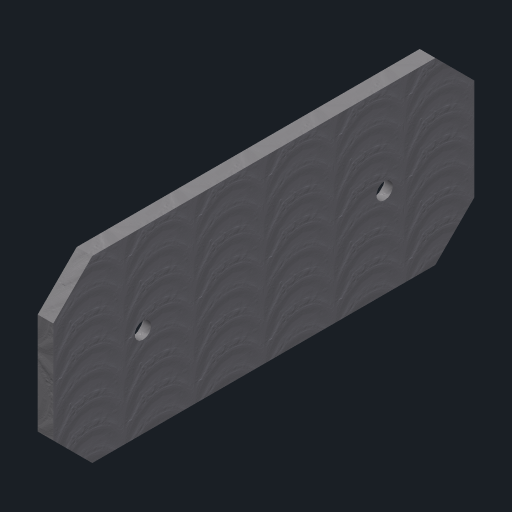
# Autodesk Inventor part: CAJA
Saved by Autodesk Inventor 2024.3 (Build 283343000, 343)
## iProperties
Created: 2024-06-29
Part Number: CAJA
Material: Steel, Mild, Welded
Document SubType Name: Modeling
Designer: Niler
Density: 7.85 g/cm^3
Appearance: Weld - Steel Mild
Author: Niler
Autodesk Inventor part; units mm, degrees
ref_plane "YZ Plane" through (0, 0, 0) normal (1, 0, 0) x (0, 1, 0)
ref_plane "XZ Plane" through (0, 0, 0) normal (0, 1, 0) x (-1, 0, 0)
ref_plane "XY Plane" through (0, 0, 0) normal (0, 0, 1) x (1, 0, 0)
sketch "Sketch1" plane through (0, 0, 0) normal (1, 0, 0) x (0, 1, 0)
  line L0 (-57.5, 135) -> (57.5, 135)
  line L1 (57.5, 135) -> (57.5, -135)
  line L2 (57.5, -135) -> (-57.5, -135)
  line L3 (-57.5, -135) -> (-57.5, 135)
  line L4 (-57.5, 135) -> (57.5, -135) construction
  line L5 (57.5, 135) -> (-57.5, -135) construction
  circle A0 centre (0, 77.5) radius 5.3
  circle A1 centre (0, -77.5) radius 5.3
  circle A2 centre (0, 0) radius 5.3
  line L6 (0, 77.5) -> (0, -77.5) construction
  line L7 (51.5, -129) -> (51.5, 129)
  line L8 (51.5, 129) -> (-51.5, 129)
  line L9 (-51.5, 129) -> (-51.5, -129)
  line L10 (-51.5, -129) -> (51.5, -129)
  dimension "d0" = 155
  dimension "d1" = 10.6
  dimension "d2" = 270
  dimension "d3" = 115
  dimension "d4" = 6
  constraints: 22 end point, 4 parallel, 3 centre point, 3 midpoint, 2 equal radius, 2 perpendicular, 2 vertical alignment, 1 coincident, 1 horizontal, 1 vertical, 3 other
  measures "d0" distance of L6.end L6.start
  measures "d1" diameter of A0
  measures "d2" distance between parallel lines of L2 L0
  measures "d3" distance of L0.start L0.end
  measures "d4" distance between parallel lines of L1 L7
extrude "Extrusion1" add sketch "Sketch1" along normal blind 10 contours L0 L1 L2 L3 | A2 | L10 L9 L8 L7
chamfer "Chamfer2" distance 25 angle 45 4 edges at (5, 57.5, -135) (5, -57.5, -135) (5, -57.5, 135) (5, 57.5, 135)
sketch "Sketch11" plane through (0, 0, 0) normal (-1, 0, 0) x (0, 0, 1)
  circle A0 centre (-77.5, 0) radius 5.3 projected
  circle A1 centre (77.5, 0) radius 5.3 projected
  circle A2 centre (-77.5, 0) radius 11.15
  circle A3 centre (77.5, 0) radius 11.15
  point P0 (0, 0)
  dimension "d41" = 22.3
  constraints: 2 centre point, 2 coincident, 1 equal radius
  measures "d41" diameter of A2
extrude "Extrusion10" cut sketch "Sketch11" against normal blind 5 contours A0 | A1 | A2 | A3
sketch "Sketch12" plane through (0, 0, 0) normal (-1, 0, 0) x (0, 0, 1)
  circle A0 centre (0, -15) radius 9.65
  point P0 (0, 0)
  dimension "d44" = 15
  dimension "d45" = 19.3
  constraints: 1 centre point, 1 vertical alignment
  measures "d44" distance of A0.centre point (0, 0)
  measures "d45" diameter of A0
extrude "Extrusion11" cut sketch "Sketch12" against normal blind 5
sketch "Sketch13" plane through (5, -15, 0) normal (-1, 0, 0) x (0, 0, 1)
  circle A0 centre (0, 0) radius 9.65 projected
  circle A1 centre (0, 0) radius 7.5
  point P0 (0, 15)
  dimension "d48" = 15
  constraints: 1 centre point, 1 coincident
  measures "d48" diameter of A1
extrude "Extrusion12" cut sketch "Sketch13" against normal blind 1 contours A1
body "Solid1"
